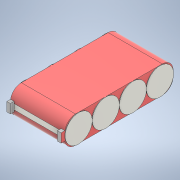
# Autodesk Inventor part: Battery_template
Saved by Autodesk Inventor 2022 (Build 260153000, 153)
## iProperties
Created: 2023-01-07
Part Number: Battery_template
Material: Generic
Document SubType Name: Modeling
Designer: Harmonic Ash
Density: 1 g/cm^3
Appearance: Default
Author: Harmonic Ash
Autodesk Inventor part; units mm, degrees
ref_plane "YZ Plane" through (0, 0, 0) normal (1, 0, 0) x (0, 1, 0)
ref_plane "XZ Plane" through (0, 0, 0) normal (0, 1, 0) x (-1, 0, 0)
sketch "Sketch1" plane through (0, 0, 0) normal (0, 1, 0) x (-1, 0, 0)
  line L0 (15, 30) -> (-15, 30)
  line L1 (-15, 30) -> (-15, -30)
  line L2 (-15, -30) -> (15, -30)
  line L3 (15, -30) -> (15, 30)
  point P0 (0, 0)
  dimension "d0" = 30
  dimension "d1" = 60
  dimension "d2" = 30
  dimension "d3" = 15
  constraints: 8 end point, 2 parallel, 1 horizontal, 1 perpendicular
  measures "d0" distance of L2.end L1.end
  measures "d1" distance of L1.end L0.end
  measures "d2" distance from line of L0 point (0, 0)
  measures "d3" distance from line of point (0, 0) L3
extrude "Extrusion1" add sketch "Sketch1" along normal blind 15
sketch "Sketch2" plane through (-15, 0, 30) normal (0, 0, 1) x (1, 0, 0)
  line L0 (0, 0) -> (0, 15) projected
  line L1 (0, 10) -> (2, 10)
  line L2 (2, 10) -> (2, 5)
  line L3 (2, 5) -> (0, 5)
  line L4 (0, 5) -> (0, 10)
  line L5 (0, 15) -> (30, 15) projected
  line L6 (30, 0) -> (30, 15) projected
  line L7 (28, 10) -> (30, 10)
  line L8 (30, 10) -> (30, 5)
  line L9 (30, 5) -> (28, 5)
  line L10 (28, 5) -> (28, 10)
  point P0 (15, 0)
  point P1 (0, 5)
  dimension "d6" = 2
  dimension "d7" = 5
  dimension "d8" = 5
  dimension "d9" = 2
  dimension "d10" = 5
  dimension "d11" = 5
  constraints: 16 end point, 4 parallel, 2 horizontal, 2 perpendicular, 2 point on line
  measures "d6" distance of L2.end L3.end
  measures "d7" distance of L1.end L2.end
  measures "d8" distance between parallel lines of L5 L1
  measures "d9" distance between parallel lines of L6 L10
  measures "d10" distance between parallel lines of L5 L7
  measures "d11" distance of L9.end L7.start
extrude "Extrusion2" add sketch "Sketch2" along normal blind 2
fillet "Fillet1" radius 6 4 edges at (0, 15, 30) (0, 0, 30) (0, 15, -30) (0, 0, -30)
sketch "Sketch3" plane through (15, 5, 32) normal (1, 0, 0) x (0, 0, -1)
  line L0 (62, 1) -> (62, 4) projected
  line L1 (62, 2.5) -> (0, 2.5)
  line L2 (0, 5) -> (0, 0) projected
  circle A0 centre (9.5, 2.5) radius 7.5
  line L3 (8, 10) -> (56, 10) projected
  circle A1 centre (24.5, 2.5) radius 7.5153
  circle A2 centre (39.5, 2.5) radius 7.5162
  circle A3 centre (54.5, 2.5) radius 7.5
  point P0 (32, -5)
  point P1 (47.0081, 2.8488)
  point P2 (47.0081, 2.1512)
  point P3 (39.9933, 10)
  point P4 (39.0067, 10)
  point P5 (31.9995, 2.9861)
  point P6 (31.9995, 2.0139)
  point P7 (24.9788, 10)
  point P8 (24.0212, 10)
  point P9 (16.9924, 2.8385)
  point P10 (16.9924, 2.1615)
  dimension "d15" = 15
  dimension "d16" = 15
  dimension "d17" = 15
  dimension "d18" = 15
  dimension "d19" = 7.5
  constraints: 4 centre point, 4 point on line, 2 end point, 2 midpoint, 1 tangent
  measures "d15" distance of A1.centre A0.centre
  measures "d16" distance of A2.centre A1.centre
  measures "d17" diameter of A3
  measures "d18" distance of A2.centre A3.centre
  measures "d19" distance of A3.centre L1.start
extrude "Extrusion3" add sketch "Sketch3" along normal blind 0.25 contours A3 A2 L1 | L1 A2 A3 | A2 A1 L1 A3 | L1 A1 A2 L3 A3 | A1 A0 L1 A2 | A0 L1 A1 | L1 A0 A1 L3 A2 | A0 A1 L1 picked at (56.9349, 1.9104) picked at (56.9427, 3.0563) picked at (7.0655, 1.9102) picked at (7.0576, 3.0563)
ref_plane "Work Plane1" through (0, 15, 22.5) normal (1, 0, 0) x (0, 0, -1)
mirror "Mirror1" about plane through (0, 15, 22.5) normal (1, 0, 0) of "Extrusion3"
equation "\"d2\" = 0.5 * d1"
equation "\"d3\" = 0.5 * d0"
body "Solid1"
